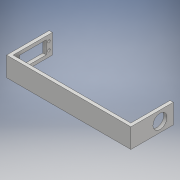
# Autodesk Inventor part: outerGantry
Saved by Autodesk Inventor 2018 (Build 220112000, 112)
## iProperties
Created: 2017-07-30
Part Number: outerGantry
Material: Generic
Document SubType Name: Modeling
Designer: kurtis
Density: 1 g/cm^3
Appearance: Default
Author: kurtis
Autodesk Inventor part; units mm, degrees
ref_plane "YZ Plane" through (0, 0, 0) normal (1, 0, 0) x (0, 1, 0)
ref_plane "XZ Plane" through (0, 0, 0) normal (0, 1, 0) x (-1, 0, 0)
ref_plane "XY Plane" through (0, 0, 0) normal (0, 0, 1) x (1, 0, 0)
sketch "Sketch1" plane through (0, 0, 0) normal (0, 0, 1) x (1, 0, 0)
  line L0 (0, 0) -> (180, 0)
  line L1 (0, 0) -> (0, 60)
  line L2 (0, 60) -> (-5, 60)
  line L3 (-5, 60) -> (-5, -5)
  line L4 (-5, -5) -> (185, -5)
  line L5 (185, -5) -> (185, 60)
  line L6 (185, 60) -> (180, 60)
  line L7 (180, 60) -> (180, 0)
  dimension "d0" = 180
  dimension "d1" = 60
  dimension "d2" = 5
  dimension "d3" = 65
  dimension "d4" = 190
  dimension "d5" = 65
  dimension "d6" = 5
  constraints: 16 end point, 3 vertical, 2 horizontal, 2 perpendicular
  measures "d0" distance of L0.start L0.end
  measures "d1" distance of L0.start L1.end
  measures "d2" distance of L1.end L2.end
  measures "d3" distance of L2.end L3.end
  measures "d4" distance of L3.end L4.end
  measures "d5" distance of L4.end L5.end
  measures "d6" distance of L5.end L6.end
extrude "Extrusion1" add sketch "Sketch1" along normal blind 30
sketch "Sketch2" plane through (-5, -5, 0) normal (-1, 0, 0) x (0, 0, 1)
  line L0 (0, 65) -> (30, 65) construction
  line L1 (15, 65) -> (15, 35) construction
  line L2 (5, 14.5) -> (25, 14.5)
  line L3 (25, 14.5) -> (25, 55.5)
  line L4 (25, 55.5) -> (5, 55.5)
  line L5 (5, 55.5) -> (5, 14.5)
  line L6 (5, 14.5) -> (25, 55.5) construction
  line L7 (25, 14.5) -> (5, 55.5) construction
  line L8 (5, 55.5) -> (5, 59.5) construction
  line L9 (5, 59.5) -> (9, 59.5) construction
  line L10 (25, 55.5) -> (25, 59.5) construction
  line L11 (25, 59.5) -> (21, 59.5) construction
  line L12 (5, 14.5) -> (5, 10.5) construction
  line L13 (5, 10.5) -> (9, 10.5) construction
  line L14 (25, 14.5) -> (25, 10.5) construction
  line L15 (25, 10.5) -> (21, 10.5) construction
  circle A0 centre (9, 59.5) radius 2
  circle A1 centre (21, 59.5) radius 2
  circle A2 centre (9, 10.5) radius 2
  circle A3 centre (21, 10.5) radius 2
  point P0 (0, 5)
  dimension "d9" = 30
  dimension "d10" = 20
  dimension "d11" = 41
  dimension "d12" = 4
  dimension "d13" = 4
  dimension "d14" = 4
  dimension "d15" = 4
  dimension "d16" = 4
  dimension "d17" = 4
  dimension "d18" = 4
  dimension "d19" = 4
  dimension "d20" = 4
  dimension "d21" = 4
  dimension "d22" = 4
  dimension "d23" = 4
  constraints: 30 end point, 5 perpendicular, 5 vertical, 4 centre point, 4 coincident, 3 midpoint, 2 parallel, 1 horizontal
  measures "d9" distance of L1.start L1.end
  measures "d10" distance of L4.end L3.end
  measures "d11" distance of L3.end L2.end
  measures "d12" distance of L4.end L8.end
  measures "d13" distance of L8.end L9.end
  measures "d14" distance of L3.end L10.end
  measures "d15" distance of L10.end L11.end
  measures "d16" distance of L2.start L12.end
  measures "d17" distance of L12.end L13.end
  measures "d18" distance of L2.end L14.end
  measures "d19" distance of L14.end L15.end
  measures "d20" diameter of A0
  measures "d21" diameter of A1
  measures "d22" diameter of A2
  measures "d23" diameter of A3
extrude "Extrusion2" cut sketch "Sketch2" against normal blind 10
sketch "Sketch3" plane through (180, 0, 0) normal (-1, 0, 0) x (0, 0, 1)
  line L0 (5, 50.5) -> (25, 50.5) construction
  line L1 (15, 50.5) -> (15, 39.5) construction
  circle A0 centre (15, 39.5) radius 10.75
  point P0 (0, 0)
  dimension "d26" = 11
  dimension "d27" = 21.5
  constraints: 2 end point, 1 centre point, 1 coincident, 1 midpoint, 1 vertical
  measures "d26" distance of L1.start L1.end
  measures "d27" diameter of A0
extrude "Extrusion3" cut sketch "Sketch3" against normal blind 14.5
equation "\"d3\" = d1 + d2"
equation "\"d4\" = d0 + 2 * d2"
equation "\"d5\" = d3"
equation "\"d6\" = d2"
equation "\"d14\" = d12"
equation "\"d15\" = d13"
equation "\"d16\" = d12"
equation "\"d17\" = d13"
equation "\"d18\" = d12"
equation "\"d19\" = d13"
body "Solid1"
